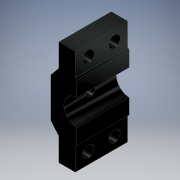
# Autodesk Inventor part: reverse gear  upper base bearing holder 1
Saved by Autodesk Inventor 2017 (Build 210142000, 142)
## iProperties
Created: 2018-11-10
Part Number: reverse gear  upper base bearing holder 1
Material: Generic
Document SubType Name: Modeling
Designer: User
Density: 1 g/cm^3
Appearance: Default
Author: User
Autodesk Inventor part; units mm, degrees
ref_plane "YZ Plane" through (0, 0, 0) normal (1, 0, 0) x (0, 1, 0)
ref_plane "XZ Plane" through (0, 0, 0) normal (0, 1, 0) x (-1, 0, 0)
ref_plane "XY Plane" through (0, 0, 0) normal (0, 0, 1) x (1, 0, 0)
sketch "Sketch1" plane through (0, 0, 0) normal (0, 1, 0) x (-1, 0, 0)
  arc A0 (0, -4) -> (0, 4) centre (0, 0) ccw
  line L0 (0, 4) -> (0, -4) construction
  line L1 (0, 4) -> (0, 9)
  line L2 (0, -4) -> (0, -9)
  line L3 (0, 9) -> (0.5, 9)
  line L4 (0.5, 9) -> (0.5, 16)
  line L5 (0, -9) -> (0.5, -9)
  line L6 (0.5, -9) -> (0.5, -16)
  line L7 (0.5, 16) -> (5.5, 16)
  line L8 (0.5, -16) -> (5.5, -16)
  line L9 (5.5, 16) -> (5.5, 9)
  line L10 (5.5, -16) -> (5.5, -9)
  line L11 (8, 0) -> (8, -6) construction
  line L12 (8, 0) -> (8, 6) construction
  line L13 (8, 6) -> (8, -6)
  line L14 (5.5, 9) -> (8, 6)
  line L15 (5.5, -9) -> (8, -6)
  dimension "d0" = 8
  dimension "d1" = 8
  dimension "d2" = 5
  dimension "d3" = 5
  dimension "d4" = 0.5
  dimension "d5" = 7
  dimension "d6" = 7
  dimension "d8" = 5
  dimension "d9" = 5
  dimension "d10" = 0
  dimension "d11" = 7
  dimension "d12" = 7
  dimension "d13" = 6
  dimension "d14" = 6
  dimension "d15" = 8
  dimension "d17" = 140.194
  constraints: 32 end point, 8 vertical, 4 horizontal, 2 point on circle, 1 centre point, 1 coincident, 1 collinear, 1 perpendicular
  measures "d0" diameter of A0
  measures "d1" distance of L0.start L0.end
  measures "d2" distance of L0.start L1.end
  measures "d3" distance of L0.end L2.end
  measures "d4" distance of L1.end L3.end
  measures "d5" distance of L3.end L4.end
  measures "d6" distance of L5.end L6.end
  measures "d8" distance of L4.end L7.end
  measures "d9" distance of L6.end L8.end
  measures "d10" distance between parallel lines of L4 L6
  measures "d11" distance of L7.end L9.end
  measures "d12" distance of L8.end L10.end
  measures "d13" distance of L11.start L11.end
  measures "d14" distance of L11.start L12.end
  measures "d15" distance between parallel lines of L12 L0
  measures "d17" angle of L9 L14
extrude "Extrusion1" add sketch "Sketch1" along normal blind 16
sketch "Sketch2" plane through (-8, 0, -6) normal (-1, 0, 0) x (0, 0, 1)
  line L0 (15, 0) -> (22, 0) projected
  line L1 (22, 0) -> (22, 16) projected
  line L2 (15, 16) -> (22, 16) projected
  line L3 (15, 0) -> (15, 16) projected
  line L4 (0, 0) -> (12, 0) projected
  line L5 (12, 0) -> (12, 16) projected
  line L6 (0, 16) -> (12, 16) projected
  line L7 (0, 0) -> (0, 16) projected
  line L8 (-10, 0) -> (-3, 0) projected
  line L9 (-3, 0) -> (-3, 16) projected
  line L10 (-10, 16) -> (-3, 16) projected
  line L11 (-10, 0) -> (-10, 16) projected
  circle A0 centre (6, 8) radius 1.5
  line L12 (4, 16) -> (12, 16)
  line L13 (8, 16) -> (20.5, 16)
  line L14 (0, 16) -> (16, 16)
  line L15 (8, 16) -> (-4.5, 16)
  line L16 (-1.3536, 16) -> (-7.8536, 16)
  line L17 (6.1, 7.993) -> (18.6, 7.993) construction
  line L18 (16.8536, 0) -> (16.8536, 16) construction
  line L19 (18.6, 7.993) -> (18.6, 3.993) construction
  line L20 (18.6, 3.993) -> (18.6, 11.993) construction
  line L21 (6.1, 7.993) -> (-6.5036, 7.993) construction
  line L22 (-6.5036, 7.993) -> (-6.5036, 3.993) construction
  line L23 (-6.5036, 3.993) -> (-6.5036, 11.993) construction
  circle A1 centre (18.6, 3.993) radius 1.75
  circle A2 centre (18.6, 11.993) radius 1.75
  circle A3 centre (-6.5036, 3.993) radius 1.75
  circle A4 centre (-6.5036, 11.993) radius 1.75
  point P0 (6, 0)
  point P1 (8, 0)
  dimension "d22" = 3
  dimension "d38" = 12.5
  dimension "d39" = 12.5
  dimension "d40" = 4
  dimension "d41" = 8
  dimension "d42" = 3.5
  dimension "d43" = 3.5
  dimension "d44" = 3.5
  dimension "d45" = 3.5
  dimension "d46" = 3.6
  dimension "d47" = 90
  dimension "d48" = 90
  dimension "d49" = 90
  dimension "d50" = 90
  dimension "d51" = 5.1464
  dimension "d52" = 28.5036
  dimension "d53" = 8.007
  dimension "d54" = 0
  dimension "d55" = 0
  dimension "d56" = 1.5
  dimension "d57" = 0
  dimension "d58" = 16
  dimension "d59" = 6
  dimension "d60" = 10
  dimension "d61" = 14
  dimension "d62" = 16
  dimension "d63" = 15.9
  dimension "d64" = 16
  dimension "d65" = 8
  dimension "d66" = 22
  dimension "d67" = 23.3535
  dimension "d68" = 4.007
  dimension "d69" = 12.007
  dimension "d70" = 29.8535
  constraints: 24 end point, 5 centre point, 4 coincident, 3 perpendicular, 3 point on line, 1 collinear, 1 horizontal, 1 midpoint, 1 parallel
  measures "d22" diameter of A0
  measures "d38" distance of L13.start L13.end
  measures "d39" distance of L13.start L15.end
  measures "d40" distance of L17.end L19.end
  measures "d41" distance of L19.end L20.end
  measures "d42" diameter of A1
  measures "d43" diameter of A2
  measures "d44" diameter of A3
  measures "d45" diameter of A4
  measures "d46" distance from line of L3 A2.centre
  measures "d47" angle of L1 L13
  measures "d48" angle of L1 L12
  measures "d49" angle of L1 L16
  measures "d50" angle of L15 L1
  measures "d51" distance between parallel lines of L1 L18
  measures "d52" distance between parallel lines of L1 L22
  measures "d53" distance between parallel lines of L2 L17
  measures "d54" distance between parallel lines of L13 L14
  measures "d55" distance from line of L1.end L13
  measures "d56" distance from line of L13.end L1
  measures "d57" distance from line of L18.end L2
  measures "d58" distance from line of L18.start L2
  measures "d59" distance from line of L14.end L1
  measures "d60" distance from line of L12.end L1
  measures "d61" distance from line of point (8, 0) L1
  measures "d62" distance from line of point (8, 0) L2
  measures "d63" distance from line of L17.start L1
  measures "d64" distance from line of A0.centre L1
  measures "d65" distance from line of A0.centre L2
  measures "d66" distance from line of L14.start L1
  measures "d67" distance from line of L16.start L1
  measures "d68" distance from line of L23.end L2
  measures "d69" distance from line of L22.end L2
  measures "d70" distance from line of L16.end L1
extrude "Extrusion3" cut sketch "Sketch2" against normal through all contours A0
chamfer "Chamfer1" distance 1 angle 45 1 edges at (-8, 8, -1.5)
chamfer "Chamfer2" distance 0.4 angle 45 2 edges at (0, 8, 9) (0, 8, -9)
extrude "Extrusion5" cut sketch "Sketch2" against normal blind 15 contours A1 | A2 | A3 | A4
body "Solid1"
